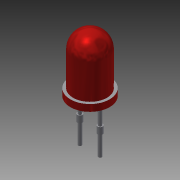
# Autodesk Inventor part: LED
Saved by Autodesk Inventor 2013 SP1 (Build 170176100, 176)
## iProperties
Created: 2012-12-07
Part Number: LED
Material: Allgemein
Document SubType Name: Modeling
Designer: Sebastian
Density: 1 g/cm^3
Author: Sebastian
Autodesk Inventor part; units mm, degrees
ref_plane "YZ Plane" through (0, 0, 0) normal (1, 0, 0) x (0, 1, 0)
ref_plane "XZ Plane" through (0, 0, 0) normal (0, 1, 0) x (-1, 0, 0)
ref_plane "XY Plane" through (0, 0, 0) normal (0, 0, 1) x (1, 0, 0)
sketch "Skizze1" plane through (0, 0, 0) normal (0, 0, 1) x (1, 0, 0)
  circle A0 centre (0, 0) radius 2.5
  dimension "d0" = 5
  constraints: 1 centre point, 1 coincident
  measures "d0" diameter of A0
extrude "Extrusion1" add sketch "Skizze1" along normal blind 7.5
fillet "Rundung1" radius 2.5 1 edges at (-2.5, 0, 7.5)
sketch "Skizze2" plane through (0, 0, 0) normal (0, 0, 1) x (1, 0, 0)
  circle A0 centre (0, 0) radius 2.9
  dimension "d4" = 5.8
  constraints: 1 centre point, 1 coincident
  measures "d4" diameter of A0
extrude "Extrusion2" add sketch "Skizze2" against normal blind 1
sketch "Skizze Helper" plane through (0, 0, 0) normal (0, 0, 1) x (1, 0, 0)
  circle A0 centre (0, 0) radius 1.5 construction
  dimension "d12" = 3
  constraints: 1 centre point
  measures "d12" diameter of A0
sketch "Skizze5" plane through (0, 0, 0) normal (0, 0, 1) x (1, 0, 0)
  circle A0 centre (-1.491, 0) radius 0.25
  point P0 (0, 0)
  dimension "d13" = 0.5
  constraints: 1 centre point
  measures "d13" diameter of A0
extrude "Extrusion Bein" add sketch "Skizze5" against normal blind 7 separate body
move or copy body "Körper verschieben Bein" bodies to move or copy 2 copy no translate (0, 0, -1)
sketch "Skizze7" plane through (0, 0, 0) normal (0, 0, 1) x (1, 0, 0)
  circle A0 centre (-1.5, 0) radius 0.375
  point P0 (0, 0)
  dimension "d23" = 0.75
  constraints: 1 centre point
  measures "d23" diameter of A0
extrude "Extrusion Lötpunkt" add sketch "Skizze7" against normal blind 1 separate body
move or copy body "Körper verschieben Lötpunkt" bodies to move or copy 3 copy no translate (0, 0, -4)
sketch "Skizze Helper2" plane through (0, 0, 0) normal (0, 1, 0) x (-1, 0, 0)
  point P0 (0, 0)
mirror "Spiegeln1" about plane through (0, 0, 0) normal (1, 0, 0) bodies 2
mirror "Spiegeln2" about plane through (0, 0, 0) normal (1, 0, 0) bodies 3
